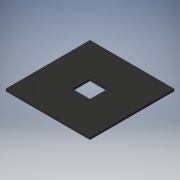
# Autodesk Inventor part: sorbothane-base-38in
Saved by Autodesk Inventor 2019 (Build 230136000, 136)
## iProperties
Created: 2019-04-16
Part Number: sorbothane-base-38in
Material: Rubber
Document SubType Name: Modeling
Designer: Wilson Lab
Density: 0.93 g/cm^3
Appearance: Rubber - Black
Author: Wilson Lab
Autodesk Inventor part; units mm, degrees
ref_plane "YZ Plane" through (0, 0, 0) normal (1, 0, 0) x (0, 1, 0)
ref_plane "XZ Plane" through (0, 0, 0) normal (0, 1, 0) x (-1, 0, 0)
ref_plane "XY Plane" through (0, 0, 0) normal (0, 0, 1) x (1, 0, 0)
sketch "Sketch1" plane through (0, 0, 0) normal (0, 1, 0) x (-1, 0, 0)
  line L0 (-177.8, 177.8) -> (177.8, 177.8)
  line L1 (177.8, 177.8) -> (177.8, -177.8)
  line L2 (177.8, -177.8) -> (-177.8, -177.8)
  line L3 (-177.8, -177.8) -> (-177.8, 177.8)
  line L4 (-177.8, 177.8) -> (177.8, -177.8) construction
  line L5 (177.8, 177.8) -> (-177.8, -177.8) construction
  line L6 (-38.1, 38.1) -> (38.1, 38.1)
  line L7 (38.1, 38.1) -> (38.1, -38.1)
  line L8 (38.1, -38.1) -> (-38.1, -38.1)
  line L9 (-38.1, -38.1) -> (-38.1, 38.1)
  line L10 (-38.1, 38.1) -> (38.1, -38.1) construction
  line L11 (38.1, 38.1) -> (-38.1, -38.1) construction
  point P0 (0, 0)
  dimension "d0" = 355.6
  dimension "d1" = 355.6
  dimension "d4" = 76.2
  constraints: 24 end point, 4 midpoint, 4 parallel, 2 horizontal, 2 perpendicular, 1 point on line
  measures "d0" distance of L0.end L1.end
  measures "d1" distance of L1.end L2.end
  measures "d4" distance of L6.end L7.end
extrude "Extrusion1" add sketch "Sketch1" along normal blind 9.525
body "Solid1"
